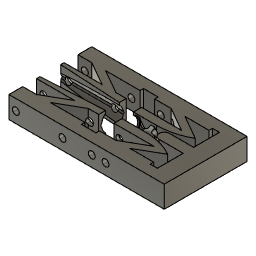
2022_09_04_Midi Spring Tin08mm Holder v2 (Autodesk Fusion 360 design; units mm, degrees)
Autodesk Fusion 360 part; units mm, degrees
sketch "Sketch1" plane through (0, 0, 0) normal (0, 1, 0) x (1, 0, 0)
  line L0 (5.5338, -2.4006) -> (2.2338, -2.4006)
  line L1 (2.2338, -5.5506) -> (0.9338, -5.5506)
  line L2 (9.5338, -2.4006) -> (9.5338, -2.9006)
  line L3 (-0.9662, -5.2602) -> (-0.9662, -5.5506)
  line L4 (5.5338, -2.4006) -> (7.2338, -2.4006)
  line L5 (0.9338, -2.4006) -> (2.2338, -2.4006)
  line L6 (6.5338, -2.4006) -> (9.5338, -2.4006)
  spline S0 degree 5 poles (2.2338, -5.5506) (2.2985, -5.4527) (2.428, -5.2649) (2.6225, -5.0076) (2.8826, -4.7141) (3.2089, -4.4353) (3.5366, -4.2528) (3.8659, -4.1745) (4.1966, -4.2053) (4.5289, -4.3414) (4.8625, -4.5749) (5.1304, -4.8334) (5.3319, -5.0651) (5.4665, -5.236) (5.5338, -5.3256) knots 0 0 0 0 0 0 0.1 0.2 0.3 0.4 0.5 0.6 0.7 0.8 0.9 1 1 1 1 1 1
  line L7 (6.5338, -5.3256) -> (9.5338, -2.9006)
  line L8 (0.9338, -2.4006) -> (-0.9662, -2.4006)
  line L9 (-0.9662, -5.2602) -> (0.9338, -5.2602)
  line L10 (-21.9662, -5.5506) -> (-0.9662, -5.5506)
  line L11 (-21.9662, -2.4006) -> (-21.9662, -5.5506)
  line L12 (0.9338, -5.2602) -> (0.9338, -5.5506)
  line L13 (6.5338, -5.3256) -> (5.5338, -5.3256)
  line L14 (-0.9662, -2.4006) -> (-21.9662, -2.4006)
revolve "Revolve1" add sketch "Sketch1" angle 360 about axis through (-0.9662, 0, 2.4006) along (-1, 0, 0) makes body 1
sketch "Sketch2" plane through (0, 0, 0) normal (0, 0, 1) x (1, 0, 0)
  line L0 (0, 0) -> (0, -2)
  line L1 (0, -2) -> (18, -2)
  line L2 (18, -2) -> (18, -4)
  line L3 (18, -4) -> (0, -4)
  line L4 (0, -4) -> (0, -2)
  line L5 (0, -8) -> (18, -8)
  line L6 (18, -8) -> (18, -10)
  line L7 (18, -10) -> (0, -10)
  line L8 (0, -10) -> (0, -8)
  line L9 (4, -8) -> (11, -4)
  line L10 (8, -8) -> (15, -4)
  line L11 (0, -3) -> (18, -2)
  circle A0 centre (0, 0) radius 0.5
  dimension "d2" = 2
  dimension "d6" = 1
  constraint vertical L0
  constraint horizontal L1
  constraint vertical L2
  constraint horizontal L3
  constraint vertical L4
  constraint horizontal L5
  constraint vertical L6
  constraint horizontal L7
  constraint vertical L8
  constraint coincident L5 L9.start
  constraint coincident L3 L9.end
  constraint coincident L5 L10.start
  constraint coincident L3 L10.end
  constraint parallel L9 L10
  constraint midpoint L4 L11.start
  constraint coincident L0.start A0.centre
  measures "d2" distance of L0.start L0.end
  measures "d6" diameter of A0
extrude "Extrude1" add sketch "Sketch2" along normal blind 3.15 and the other way blind 3.15 separate body contours L2 L3 L4 L11 | L3 L5 L9 L10 | L5 L6 L7 L8 makes body 2
sketch "Sketch3" plane through (0, 0, 0) normal (0, 0, 1) x (1, 0, 0)
  circle A0 centre (0, 0) radius 0.5
  dimension "d5" = 1
  constraint coincident A0.centre origin
  measures "d5" diameter of A0
move_body "Move1" bodies 1 to x (1, 0, 0) y (0, 1, 0) z (0, 0, 1) at (21.9662, 0, -2.4006)
combine "Combine1" operation cut target body 2 tool bodies 1 keep tools
sketch "Sketch4" plane through (0, 0, 0) normal (1, 0, 0) x (0, 1, 0)
  line L0 (0, 0) -> (-3, 0)
  circle A0 centre (-3, 0) radius 0.4
  dimension "d9" = 3
  dimension "d10" = 0.8
  constraint coincident L0.start origin
  constraint horizontal L0
  constraint coincident L0.end A0.centre
  measures "d9" distance of L0.start L0.end
  measures "d10" diameter of A0
extrude "Extrude2" cut sketch "Sketch4" along normal blind 18 bodies 2
sketch "Sketch5" plane through (0, 0, 0) normal (0, 1, 0) x (1, 0, 0)
  circle A0 centre (2, 0) radius 1
  circle A1 centre (15.5, 0) radius 1
  dimension "d13" = 2
  dimension "d14" = 2
  measures "d13" diameter of A0
  measures "d14" diameter of A1
extrude "Extrude3" cut sketch "Sketch5" against normal blind 17.5 bodies 2
sketch "Sketch6" plane through (0, 0, 0) normal (0, 0, 1) x (1, 0, 0)
  line L0 (37.9612, -10) -> (22.2158, -10)
  line L1 (22.2158, -10) -> (22.2158, -8)
  line L2 (22.2158, -8) -> (37.9612, -8)
  line L3 (37.9612, -8) -> (37.9612, -10)
  line L4 (31, -8) -> (38, -4)
  line L5 (27, -8) -> (34, -4)
  line L6 (33.5669, 3.6069) -> (33.5669, -4) construction
  line L7 (22.4267, -4) -> (34, -4)
  line L8 (22.4267, -4) -> (29.1505, -4)
  line L9 (29.1505, -4) -> (29.1505, -1.647)
  line L10 (29.1505, -1.647) -> (22.4267, -1.647)
  line L11 (22.4267, -1.647) -> (22.4267, -4)
  arc A0 (38, -4) -> (29.1505, -1.647) centre (29.1505, -19.4649) ccw
  constraint horizontal L2
  constraint vertical L3
  constraint horizontal L0
  constraint vertical L1
  constraint coincident L5.start L2
  constraint coincident L4.start L2
  constraint parallel L4 L5
  constraint horizontal L7
  constraint horizontal L8
  constraint vertical L9
  constraint horizontal L10
  constraint vertical L11
  constraint tangent L10 A0
extrude "Extrude4" add sketch "Sketch6" along normal blind 3.15 and the other way blind 3.15 separate body makes body 3
combine "Combine2" operation cut target body 3 tool bodies 1 keep tools
sketch "Sketch7" plane through (0, 0, 0) normal (0, 1, 0) x (1, 0, 0)
  circle A0 centre (24, 0) radius 1
  circle A1 centre (28, 0) radius 1
extrude "Extrude5" cut sketch "Sketch7" against normal blind 15 bodies 3
sketch "Sketch8" plane through (0, 0, 0) normal (1, 0, 0) x (0, 1, 0)
copy_body "CopyPasteBodies1" bodies 2 3 makes body 4 makes body 5
move_body "Move2" bodies 4 5 to x (1, 0, 0) y (0, -1, 0) z (0, 0, -1) at (0, 0, 0)
sketch "Sketch9" plane through (0, 0, 0) normal (0, 0, 1) x (1, 0, 0)
  line L0 (0, 12) -> (40, 12)
  line L1 (40, 12) -> (40, 9)
  line L2 (40, 9) -> (0, 9)
  line L3 (0, 9) -> (0, 12)
  line L4 (33, 1.5) -> (40, 1.5)
  line L5 (40, 1.5) -> (40, -1.5)
  line L6 (40, -1.5) -> (33, -1.5)
  line L7 (40, 12) -> (45, 12)
  line L8 (45, 12) -> (45, -12)
  line L9 (45, -12) -> (40, -12)
  line L10 (40, -12) -> (40, 12)
  line L11 (40, -12) -> (0, -12)
  line L12 (0, -12) -> (0, -9)
  line L13 (0, -9) -> (40, -9)
  line L14 (40, -9) -> (40, -12)
  circle A0 centre (33, 0) radius 1.5
  constraint horizontal L0
  constraint vertical L1
  constraint horizontal L2
  constraint vertical L3
  constraint horizontal L4
  constraint vertical L5
  constraint horizontal L6
  constraint horizontal L7
  constraint vertical L8
  constraint horizontal L9
  constraint vertical L10
  constraint horizontal L11
  constraint vertical L12
  constraint horizontal L13
  constraint vertical L14
  constraint coincident A0 L4.start
  constraint coincident A0 L6.end
extrude "Extrude6" add sketch "Sketch9" along normal blind 3.15 and the other way blind 3.15 bodies 2 3 4 5
extrude "Extrude7" cut sketch "Sketch7" along normal blind 21 and the other way blind 21 bodies 2
extrude "Extrude8" cut sketch "Sketch5" along normal blind 18 and the other way blind 25 bodies 2
hidden bodies 1
equation "d3 = 6.3 mm / 2"
equation "d7 = 6.3 mm / 2"
named bodies: "MidiJack63", "CableSpring", "CableSpring (1)"
